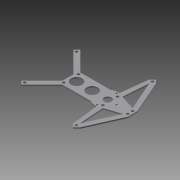
# Autodesk Inventor part: Bearing Plate
Saved by Autodesk Inventor 2013 (Build 170138000, 138)
## iProperties
Created: 2013-01-16
Part Number: Bearing Plate
Material: Generic
Document SubType Name: Modeling
Designer: actoennies
Density: 1 g/cm^3
Mass: 36.8738 g
Surface Area: 290.105 cm^2
Volume: 36.8738 cm^3
Author: actoennies
Autodesk Inventor part; units mm, degrees
ref_plane "YZ Plane" through (0, 0, 0) normal (1, 0, 0) x (0, 1, 0)
ref_plane "XZ Plane" through (0, 0, 0) normal (0, 1, 0) x (-1, 0, 0)
ref_plane "XY Plane" through (0, 0, 0) normal (0, 0, 1) x (1, 0, 0)
sketch "Sketch1" plane through (0, 0, 0) normal (0, 1, 0) x (-1, 0, 0)
  line L0 (0, 0) -> (-114.3, 0)
  line L1 (-114.3, 0) -> (-114.3, 50.8)
  line L2 (-114.3, 50.8) -> (0, 50.8)
  line L3 (0, 50.8) -> (0, 0)
  circle A0 centre (-101.6, 25.4) radius 9.5
  circle A1 centre (-60.96, 25.4) radius 14.2875
  circle A2 centre (-20.32, 25.4) radius 14.2875
  dimension "d3" = 50.8
  dimension "d4" = 19
  dimension "d12" = 28.575
  dimension "d13" = 40.64
  dimension "d14" = 114.3
  dimension "d15" = 28.575
  dimension "d16" = 40.64
  dimension "d56" = 20.32
  dimension "d57" = 25.4
  dimension "d58" = 25.4
  dimension "d59" = 25.4
  constraints: 8 end point, 3 centre point, 2 parallel, 1 horizontal, 1 perpendicular
  measures "d3" distance of L2.end L0.start
  measures "d4" diameter of A0
  measures "d12" diameter of A1
  measures "d13" distance of A1.centre A0.centre
  measures "d14" distance of L0.start L0.end
  measures "d15" diameter of A2
  measures "d16" distance of A2.centre A1.centre
  measures "d56" distance from line of L3 A2.centre
  measures "d57" distance from line of L0 A2.centre
  measures "d58" distance from line of A1.centre L0
  measures "d59" distance from line of L0 A0.centre
extrude "Extrusion3" add sketch "Sketch1" along normal blind 3.175
sketch "Sketch2" plane through (0, 3.175, 0) normal (0, 1, 0) x (1, 0, 0)
  line L0 (114.3, 0) -> (0, 0) projected
  line L1 (0, -50.8) -> (114.3, -50.8) projected
  line L2 (114.3, -50.8) -> (114.3, 0) projected
  circle A0 centre (107.95, -6.35) radius 3.3782
  circle A1 centre (107.95, -44.45) radius 3.3782
  dimension "d19" = 6.7564
  dimension "d20" = 6.7564
  dimension "d21" = 6.35
  dimension "d22" = 6.35
  dimension "d23" = 6.35
  dimension "d24" = 6.35
  constraints: 2 centre point
  measures "d19" diameter of A0
  measures "d20" diameter of A1
  measures "d21" distance from line of L0 A0.centre
  measures "d22" distance from line of L2 A0.centre
  measures "d23" distance from line of L2 A1.centre
  measures "d24" distance from line of L1 A1.centre
extrude "Extrusion4" cut sketch "Sketch2" against normal blind 25.4
sketch "Sketch3" plane through (0, 3.175, 0) normal (0, 1, 0) x (1, 0, 0)
  line L0 (114.3, 0) -> (0, 0) projected
  line L1 (0, 0) -> (0, -50.8) projected
  line L2 (0, -50.8) -> (114.3, -50.8) projected
  circle A0 centre (6.35, -6.35) radius 3.3782
  circle A1 centre (6.35, -44.45) radius 3.3782
  dimension "d27" = 6.7564
  dimension "d28" = 6.7564
  dimension "d29" = 6.35
  dimension "d30" = 6.35
  dimension "d31" = 6.35
  dimension "d32" = 6.35
  constraints: 2 centre point
  measures "d27" diameter of A0
  measures "d28" diameter of A1
  measures "d29" distance from line of L2 A1.centre
  measures "d30" distance from line of L1 A1.centre
  measures "d31" distance from line of L0 A0.centre
  measures "d32" distance from line of L1 A0.centre
extrude "Extrusion5" cut sketch "Sketch3" against normal blind 25.4
sketch "Sketch4" plane through (0, 3.175, 0) normal (0, 1, 0) x (1, 0, 0)
  circle A0 centre (6.35, -6.35) radius 3.3782 projected
  circle A1 centre (6.35, -44.45) radius 3.3782 projected
  line L0 (114.3, 0) -> (0, 0) projected
  line L1 (0, 0) -> (0, -50.8) projected
  line L2 (0, -50.8) -> (114.3, -50.8) projected
  line L3 (226.8659, 306.8695) -> (559.1354, -25.4) projected
  line L4 (559.1354, -25.4) -> (226.8659, -357.6695) projected
  line L5 (226.8659, -357.6695) -> (-105.4036, -25.4) projected
  line L6 (-105.4036, -25.4) -> (226.8659, 306.8695) projected
  circle A2 centre (-105.9649, -16.981) radius 3.3782 projected
  circle A3 centre (-97.5459, -8.562) radius 3.3782 projected
  circle A4 centre (-89.1269, -0.143) radius 3.3782 projected
  circle A5 centre (-80.7079, 8.276) radius 3.3782 projected
  circle A6 centre (-72.2889, 16.695) radius 3.3782 projected
  circle A7 centre (-63.8699, 25.1139) radius 3.3782 projected
  circle A8 centre (-55.4509, 33.5329) radius 3.3782 projected
  circle A9 centre (-47.0319, 41.9519) radius 3.3782 projected
  circle A10 centre (-39.2063, 49.7776) radius 3.3782 projected
  circle A11 centre (-31.3806, 57.6032) radius 3.3782 projected
  circle A12 centre (-23.555, 65.4289) radius 3.3782 projected
  circle A13 centre (-15.7293, 73.2545) radius 3.3782 projected
  circle A14 centre (-7.9037, 81.0802) radius 3.3782 projected
  circle A15 centre (-0.078, 88.9058) radius 3.3782 projected
  circle A16 centre (7.7476, 96.7315) radius 3.3782 projected
  circle A17 centre (15.5733, 104.5571) radius 3.3782 projected
  circle A18 centre (23.3989, 112.3828) radius 3.3782 projected
  circle A19 centre (31.2246, 120.2084) radius 3.3782 projected
  circle A20 centre (39.0502, 128.0341) radius 3.3782 projected
  circle A21 centre (46.8759, 135.8597) radius 3.3782 projected
  circle A22 centre (54.7016, 143.6854) radius 3.3782 projected
  circle A23 centre (62.5272, 151.511) radius 3.3782 projected
  circle A24 centre (70.3529, 159.3367) radius 3.3782 projected
  circle A25 centre (78.1785, 167.1623) radius 3.3782 projected
  circle A26 centre (86.0042, 174.988) radius 3.3782 projected
  circle A27 centre (93.8298, 182.8137) radius 3.3782 projected
  circle A28 centre (101.6555, 190.6393) radius 3.3782 projected
  circle A29 centre (109.4811, 198.465) radius 3.3782 projected
  circle A30 centre (117.3068, 206.2906) radius 3.3782 projected
  circle A31 centre (125.1324, 214.1163) radius 3.3782 projected
  circle A32 centre (132.9581, 221.9419) radius 3.3782 projected
  circle A33 centre (140.7837, 229.7676) radius 3.3782 projected
  circle A34 centre (148.6094, 237.5932) radius 3.3782 projected
  circle A35 centre (156.435, 245.4189) radius 3.3782 projected
  circle A36 centre (164.2607, 253.2445) radius 3.3782 projected
  circle A37 centre (172.0863, 261.0702) radius 3.3782 projected
  circle A38 centre (179.912, 268.8958) radius 3.3782 projected
  circle A39 centre (187.7376, 276.7215) radius 3.3782 projected
  circle A40 centre (195.5633, 284.5471) radius 3.3782 projected
  circle A41 centre (203.3889, 292.3728) radius 3.3782 projected
  circle A42 centre (211.2146, 300.1984) radius 3.3782 projected
  circle A43 centre (219.0402, 308.0241) radius 3.3782 projected
  circle A44 centre (226.8659, 315.8497) radius 3.3782 projected
  circle A45 centre (-114.3838, -25.4) radius 3.3782 projected
  circle A46 centre (-107.4196, -32.3643) radius 3.3782 projected
  circle A47 centre (-100.4553, -39.3286) radius 3.3782 projected
  circle A48 centre (-93.491, -46.2928) radius 3.3782 projected
  circle A49 centre (-86.5267, -53.2571) radius 3.3782 projected
  circle A50 centre (-79.5624, -60.2214) radius 3.3782 projected
  circle A51 centre (-72.5982, -67.1857) radius 3.3782 projected
  circle A52 centre (-65.6339, -74.15) radius 3.3782 projected
  circle A53 centre (-58.6696, -81.1142) radius 3.3782 projected
  circle A54 centre (-51.7053, -88.0785) radius 3.3782 projected
  circle A55 centre (-44.741, -95.0428) radius 3.3782 projected
  circle A56 centre (-37.7768, -102.0071) radius 3.3782 projected
  circle A57 centre (-30.8125, -108.9714) radius 3.3782 projected
  circle A58 centre (-23.8482, -115.9356) radius 3.3782 projected
  circle A59 centre (-16.8839, -122.8999) radius 3.3782 projected
  circle A60 centre (-9.9196, -129.8642) radius 3.3782 projected
  circle A61 centre (-2.9554, -136.8285) radius 3.3782 projected
  circle A62 centre (4.0089, -143.7928) radius 3.3782 projected
  circle A63 centre (10.9732, -150.757) radius 3.3782 projected
  circle A64 centre (17.9375, -157.7213) radius 3.3782 projected
  circle A65 centre (24.9018, -164.6856) radius 3.3782 projected
  circle A66 centre (31.866, -171.6499) radius 3.3782 projected
  circle A67 centre (38.8303, -178.6142) radius 3.3782 projected
  circle A68 centre (45.7946, -185.5784) radius 3.3782 projected
  circle A69 centre (52.7589, -192.5427) radius 3.3782 projected
  circle A70 centre (59.7232, -199.507) radius 3.3782 projected
  circle A71 centre (66.6874, -206.4713) radius 3.3782 projected
  circle A72 centre (73.6517, -213.4356) radius 3.3782 projected
  circle A73 centre (80.616, -220.3998) radius 3.3782 projected
  circle A74 centre (87.5803, -227.3641) radius 3.3782 projected
  circle A75 centre (94.5446, -234.3284) radius 3.3782 projected
  circle A76 centre (101.5088, -241.2927) radius 3.3782 projected
  circle A77 centre (108.4731, -248.257) radius 3.3782 projected
  circle A78 centre (115.4374, -255.2212) radius 3.3782 projected
  circle A79 centre (122.4017, -262.1855) radius 3.3782 projected
  circle A80 centre (129.366, -269.1498) radius 3.3782 projected
  circle A81 centre (136.3302, -276.1141) radius 3.3782 projected
  circle A82 centre (143.2945, -283.0784) radius 3.3782 projected
  circle A83 centre (150.2588, -290.0426) radius 3.3782 projected
  circle A84 centre (157.2231, -297.0069) radius 3.3782 projected
  circle A85 centre (164.1874, -303.9712) radius 3.3782 projected
  circle A86 centre (171.1516, -310.9355) radius 3.3782 projected
  circle A87 centre (178.1159, -317.8998) radius 3.3782 projected
  circle A88 centre (185.0802, -324.8641) radius 3.3782 projected
  circle A89 centre (192.0445, -331.8283) radius 3.3782 projected
  circle A90 centre (199.0088, -338.7926) radius 3.3782 projected
  circle A91 centre (205.9731, -345.7569) radius 3.3782 projected
  circle A92 centre (212.9373, -352.7212) radius 3.3782 projected
  circle A93 centre (219.9016, -359.6855) radius 3.3782 projected
  circle A94 centre (302.0435, 240.6722) radius 3.3782 projected
  circle A95 centre (309.8691, 232.8465) radius 3.3782 projected
  circle A96 centre (317.6948, 225.0209) radius 3.3782 projected
  circle A97 centre (325.5204, 217.1952) radius 3.3782 projected
  circle A98 centre (333.3461, 209.3696) radius 3.3782 projected
  circle A99 centre (341.1717, 201.5439) radius 3.3782 projected
  circle A100 centre (348.9974, 193.7182) radius 3.3782 projected
  circle A101 centre (356.823, 185.8926) radius 3.3782 projected
  circle A102 centre (364.6487, 178.0669) radius 3.3782 projected
  circle A103 centre (372.4743, 170.2413) radius 3.3782 projected
  circle A104 centre (380.3, 162.4156) radius 3.3782 projected
  circle A105 centre (388.1256, 154.59) radius 3.3782 projected
  circle A106 centre (395.9513, 146.7643) radius 3.3782 projected
  circle A107 centre (403.7769, 138.9387) radius 3.3782 projected
  circle A108 centre (411.6026, 131.113) radius 3.3782 projected
  circle A109 centre (419.4282, 123.2874) radius 3.3782 projected
  circle A110 centre (427.2539, 115.4617) radius 3.3782 projected
  circle A111 centre (435.0795, 107.6361) radius 3.3782 projected
  circle A112 centre (442.9052, 99.8104) radius 3.3782 projected
  circle A113 centre (450.7308, 91.9848) radius 3.3782 projected
  circle A114 centre (458.5565, 84.1591) radius 3.3782 projected
  circle A115 centre (466.3822, 76.3335) radius 3.3782 projected
  circle A116 centre (474.2078, 68.5078) radius 3.3782 projected
  circle A117 centre (482.0335, 60.6822) radius 3.3782 projected
  circle A118 centre (489.8591, 52.8565) radius 3.3782 projected
  circle A119 centre (497.6848, 45.0309) radius 3.3782 projected
  circle A120 centre (505.5104, 37.2052) radius 3.3782 projected
  circle A121 centre (513.3361, 29.3796) radius 3.3782 projected
  circle A122 centre (521.1617, 21.5539) radius 3.3782 projected
  circle A123 centre (528.9874, 13.7283) radius 3.3782 projected
  circle A124 centre (536.813, 5.9026) radius 3.3782 projected
  circle A125 centre (544.6387, -1.923) radius 3.3782 projected
  circle A126 centre (552.4643, -9.7487) radius 3.3782 projected
  circle A127 centre (560.29, -17.5743) radius 3.3782 projected
  circle A128 centre (568.1156, -25.4) radius 3.3782 projected
  circle A129 centre (560.29, -33.2257) radius 3.3782 projected
  circle A130 centre (552.4643, -41.0513) radius 3.3782 projected
  circle A131 centre (544.6387, -48.877) radius 3.3782 projected
  circle A132 centre (536.813, -56.7026) radius 3.3782 projected
  circle A133 centre (528.9874, -64.5283) radius 3.3782 projected
  circle A134 centre (521.1617, -72.3539) radius 3.3782 projected
  circle A135 centre (513.3361, -80.1796) radius 3.3782 projected
  circle A136 centre (505.5104, -88.0052) radius 3.3782 projected
  circle A137 centre (497.6848, -95.8309) radius 3.3782 projected
  circle A138 centre (489.8591, -103.6565) radius 3.3782 projected
  circle A139 centre (482.0335, -111.4822) radius 3.3782 projected
  circle A140 centre (474.2078, -119.3078) radius 3.3782 projected
  circle A141 centre (466.3822, -127.1335) radius 3.3782 projected
  circle A142 centre (458.5565, -134.9591) radius 3.3782 projected
  circle A143 centre (450.7308, -142.7848) radius 3.3782 projected
  circle A144 centre (442.9052, -150.6104) radius 3.3782 projected
  circle A145 centre (435.0795, -158.4361) radius 3.3782 projected
  circle A146 centre (427.2539, -166.2617) radius 3.3782 projected
  circle A147 centre (419.4282, -174.0874) radius 3.3782 projected
  circle A148 centre (411.6026, -181.913) radius 3.3782 projected
  circle A149 centre (403.7769, -189.7387) radius 3.3782 projected
  circle A150 centre (395.9513, -197.5643) radius 3.3782 projected
  circle A151 centre (388.1256, -205.39) radius 3.3782 projected
  circle A152 centre (380.3, -213.2156) radius 3.3782 projected
  circle A153 centre (372.4743, -221.0413) radius 3.3782 projected
  circle A154 centre (364.6487, -228.8669) radius 3.3782 projected
  circle A155 centre (356.823, -236.6926) radius 3.3782 projected
  circle A156 centre (348.9974, -244.5182) radius 3.3782 projected
  circle A157 centre (341.1717, -252.3439) radius 3.3782 projected
  circle A158 centre (333.3461, -260.1696) radius 3.3782 projected
  circle A159 centre (325.5204, -267.9952) radius 3.3782 projected
  circle A160 centre (317.6948, -275.8209) radius 3.3782 projected
  circle A161 centre (309.8691, -283.6465) radius 3.3782 projected
  circle A162 centre (302.0435, -291.4722) radius 3.3782 projected
  circle A163 centre (287.4826, 255.233) radius 3.3782 projected
  circle A164 centre (274.0122, 268.7034) radius 3.3782 projected
  circle A165 centre (260.5419, 282.1738) radius 3.3782 projected
  circle A166 centre (247.0715, 295.6442) radius 3.3782 projected
  circle A167 centre (233.6011, 309.1145) radius 3.3782 projected
  circle A168 centre (294.2178, 248.4978) radius 3.3782 projected
  circle A169 centre (240.3363, 302.3793) radius 3.3782 projected
  circle A170 centre (253.8067, 288.909) radius 3.3782 projected
  circle A171 centre (267.277, 275.4386) radius 3.3782 projected
  circle A172 centre (280.7474, 261.9682) radius 3.3782 projected
  circle A173 centre (268.9608, -324.5548) radius 3.3782 projected
  circle A174 centre (226.8659, -366.6497) radius 3.3782 projected
  circle A175 centre (235.2849, -358.2307) radius 3.3782 projected
  circle A176 centre (243.7039, -349.8118) radius 3.3782 projected
  circle A177 centre (252.1229, -341.3928) radius 3.3782 projected
  circle A178 centre (260.5419, -332.9738) radius 3.3782 projected
  circle A179 centre (277.3798, -316.1358) radius 3.3782 projected
  circle A180 centre (285.7988, -307.7168) radius 3.3782 projected
  circle A181 centre (294.2178, -299.2978) radius 3.3782 projected
  line L7 (226.8659, -375.63) -> (-123.3641, -25.4) projected
  line L8 (577.0959, -25.4) -> (226.8659, -375.63) projected
  line L9 (226.8659, 324.83) -> (577.0959, -25.4) projected
  line L10 (-123.3641, -25.4) -> (226.8659, 324.83) projected
  line L11 (8.9803, -50.8) -> (-44.4919, -104.2722)
  line L12 (4.4901, 0) -> (-46.737, 51.2271)
  line L13 (0, -41.8197) -> (-53.4722, -95.2919)
  line L14 (0, -13.4704) -> (-55.7172, 42.2469)
  line L15 (-53.4722, -95.2919) -> (-44.4919, -104.2722)
  line L16 (8.9803, -50.8) -> (0, -50.8)
  line L17 (0, -50.8) -> (0, -41.8197)
  line L18 (-55.7172, 42.2469) -> (-46.737, 51.2271)
  line L19 (0, -13.4704) -> (0, 0)
  line L20 (4.4901, 0) -> (0, 0)
  dimension "d35" = 6.35
  dimension "d36" = 3.175
  dimension "d39" = 12.7
  dimension "d40" = 12.7
  constraints: 20 end point, 7 point on line, 4 collinear, 4 perpendicular, 2 parallel
  measures "d35" distance from line of A1.centre L11
  measures "d36" distance from line of A0.centre L12
  measures "d39" distance between parallel lines of L13 L11
  measures "d40" distance between parallel lines of L12 L14
extrude "Extrusion6" add sketch "Sketch4" against normal blind 3.175 contours L0 L1 L14 L6 L12 | L6 L14 L10 L12 | L1 L2 L11 L5 L13 | L5 L11 A56 L7 L13 | L11 A56 picked at (-40.1488, -99.8322)
sketch "Sketch5" plane through (0, 0, 0) normal (0, -1, 0) x (1, 0, 0)
  line L0 (4.4901, 0) -> (114.3, 0) projected
  line L1 (114.3, 0) -> (114.3, 50.8) projected
  line L2 (114.3, 50.8) -> (8.9803, 50.8) projected
  arc A0 (82.793, 0) -> (82.793, 50.8) centre (99.06, 25.4) ccw
  point P0 (0, 0)
  dimension "d47" = 60.325
  constraints: 2 point on circle, 2 point on line, 1 centre point
  measures "d47" diameter of A0
extrude "Extrusion7" add sketch "Sketch5" against normal blind 3.175
sketch "Sketch6" plane through (0, 0, 0) normal (0, -1, 0) x (1, 0, 0)
  circle A0 centre (99.06, 50.8) radius 2.032
  circle A1 centre (99.06, 0) radius 2.032
  circle A2 centre (124.46, 25.4) radius 2.032
  point P0 (0, 0)
  dimension "d51" = 4.064
  dimension "d52" = 4.064
  dimension "d53" = 4.064
  constraints: 3 centre point
  measures "d51" diameter of A0
  measures "d52" diameter of A1
  measures "d53" diameter of A2
extrude "Extrusion8" cut sketch "Sketch6" against normal blind 3.175
sketch "Sketch7" plane through (0, 3.175, 0) normal (0, 1, 0) x (1, 0, 0)
  circle A0 centre (124.46, -25.4) radius 2.032 projected
  circle A1 centre (107.95, -6.35) radius 3.3782 projected
  circle A2 centre (107.95, -44.45) radius 3.3782 projected
  line L0 (114.3, -50.8) -> (153.5256, -38.1) projected
  line L1 (153.5256, -38.1) -> (119.1028, -115.2026) projected
  line L2 (119.1028, -115.2026) -> (114.3, -50.8) projected
  line L3 (153.5256, -12.7) -> (114.3, 0) projected
  line L4 (114.3, 0) -> (119.1028, 64.4026) projected
  line L5 (119.1028, 64.4026) -> (153.5256, -12.7) projected
  circle A3 centre (107.95, -44.45) radius 3.3782 projected
  circle A4 centre (107.95, -6.35) radius 3.3782 projected
  circle A5 centre (119.1028, -124.1828) radius 3.3782 projected
  circle A6 centre (159.8756, -19.05) radius 3.3782 projected
  circle A7 centre (159.8756, -31.75) radius 3.3782 projected
  circle A8 centre (119.1028, 73.3828) radius 3.3782 projected
  line L6 (101.6, -50.8) -> (110.1226, -124.1828) projected
  line L7 (110.1226, -124.1828) -> (119.1028, -133.1631) projected
  line L8 (119.1028, -133.1631) -> (128.0831, -124.1828) projected
  line L9 (128.0831, -124.1828) -> (166.2256, -38.1) projected
  line L10 (166.2256, -38.1) -> (166.2256, -12.7) projected
  line L11 (166.2256, -12.7) -> (128.0831, 73.3828) projected
  line L12 (128.0831, 73.3828) -> (119.1028, 82.3631) projected
  line L13 (119.1028, 82.3631) -> (110.1226, 73.3828) projected
  line L14 (110.1226, 73.3828) -> (101.6, 0) projected
  line L15 (101.6, 0) -> (101.6, -9.7295) projected
  arc A9 (101.6, -41.0705) -> (101.6, -9.7295) centre (99.06, -25.4) ccw projected
  line L16 (101.6, -41.0705) -> (101.6, -50.8) projected
  point P0 (0, 0)
extrude "Extrusion9" add sketch "Sketch7" against normal blind 3.175
body "Solid3"
